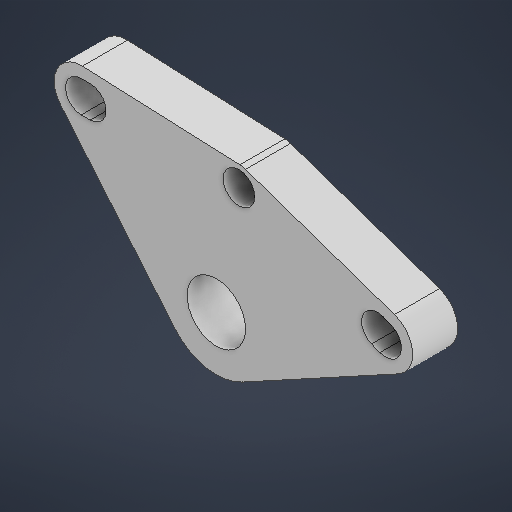
# Autodesk Inventor part: CoinLockOpener
Saved by Autodesk Inventor 2026.3 (Build 303398000, 398)
## iProperties
Created: 2026-05-05
Part Number: CoinLockOpener
Material: Generic
Document SubType Name: Modeling
Designer: frede
Density: 1 g/cm^3
Appearance: Default
Author: frede
Autodesk Inventor part; units mm, degrees
ref_plane "YZ Plane" through (0, 0, 0) normal (1, 0, 0) x (0, 1, 0)
ref_plane "XZ Plane" through (0, 0, 0) normal (0, 1, 0) x (-1, 0, 0)
ref_plane "XY Plane" through (0, 0, 0) normal (0, 0, 1) x (1, 0, 0)
sketch "Sketch1" plane through (0, 0, 0) normal (0, 0, 1) x (1, 0, 0)
  circle A0 centre (0, 0) radius 1.75
  arc A1 (-16.5, -1.75) -> (-16.5, 1.75) centre (-16.5, 0) ccw
  arc A2 (-17.5, 1.75) -> (-17.5, -1.75) centre (-17.5, 0) ccw
  line L0 (-17.5, 1.75) -> (-16.5, 1.75)
  line L1 (-17.5, -1.75) -> (-16.5, -1.75)
  arc A3 (15.9971, -4.4051) -> (14.7172, -7.6627) centre (15.3572, -6.0339) ccw
  arc A4 (15.6479, -8.0283) -> (16.9279, -4.7708) centre (16.2879, -6.3996) ccw
  line L2 (15.6479, -8.0283) -> (14.7172, -7.6627)
  line L3 (16.9279, -4.7708) -> (15.9971, -4.4051)
  circle A5 centre (16.2879, -6.3996) radius 3
  circle A6 centre (-17.5, 0) radius 3
  circle A7 centre (0, 0) radius 2.25
  line L4 (-17.3714, 2.9972) -> (0.0964, 2.2479)
  line L5 (17.2643, -3.5629) -> (0.7323, 2.1275)
  line L6 (-17.6714, -2.9951) -> (-2.0561, -3.8889)
  line L7 (15.3522, -9.2499) -> (0.4916, -4.3714)
  arc A8 (0.4916, -4.3714) -> (-2.0561, -3.8889) centre (-2.6275, -13.8725) ccw
  circle A9 centre (-2.5071, -13.2368) radius 3.25
  circle A10 centre (-2.5071, -13.2368) radius 6
  line L8 (-19.8004, -1.9257) -> (-7.1079, -17.0881)
  line L9 (17.7248, -9.0331) -> (0.3666, -18.5038)
  dimension "d0" = 3.5
  dimension "d1" = 3.5
  dimension "d2" = 3.5
  dimension "d5" = 158.55
  dimension "d7" = 6
  dimension "d9" = 6
  dimension "d10" = 4.5
  dimension "d11" = 10
  dimension "d14" = 0
  dimension "d15" = 0
  dimension "d18" = 6.5
  dimension "d19" = 12
  dimension "d20" = 20
  dimension "d21" = 20
  constraints: 20 end point, 20 point on circle, 15 tangent, 11 centre point, 5 coincident, 2 horizontal, 11 other
  measures "d0" diameter of A0
  measures "d1" diameter of A1
  measures "d2" diameter of A2
  measures "d7" diameter of A5
  measures "d9" diameter of A6
  measures "d10" diameter of A7
  measures "d11" radius of A8
  measures "d14" distance of point (0, 0) A7.centre
  measures "d15" distance of point (0, 0) A7.centre
  measures "d18" diameter of A9
  measures "d19" diameter of A10
  measures "d20" distance of A9.centre A2.centre
  measures "d21" distance of A4.centre A9.centre
extrude "Extrusion1" add sketch "Sketch1" along normal blind 5
body "Solid1"
